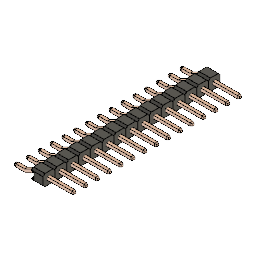
PinHeader_Male_RA_2.54mm (Autodesk Fusion 360 design; units mm, degrees)
part number: 2025-10-16-17-28-49-516
Autodesk Fusion 360 part; units mm, degrees
sketch "Sketch1" plane through (0, 0, 0) normal (0, 1, 0) x (1, 0, 0)
  line L0 (0, -0.64) -> (2.3, -0.64)
  line L1 (2.3, -0.64) -> (4.3, -1.59)
  line L2 (4.3, -1.59) -> (12.8, -1.59)
  line L3 (0, 0) -> (2.4443, 0)
  line L4 (2.4443, 0) -> (4.4443, -0.95)
  line L5 (4.4443, -0.95) -> (12.8, -0.95)
  line L6 (0, -0.64) -> (0, 0)
  line L7 (12.8, -1.59) -> (12.8, -0.95)
  line L8 (12.8, -1.27) -> (11.4, -1.27)
  dimension "d1" = 0.64
  dimension "d2" = 2.3
  dimension "d3" = 2
  dimension "d4" = 8.5
  dimension "d5" = -0.64
  dimension "d26" = 1.27
  constraint horizontal L0
  constraint parallel L0 L2
  constraint coincident L3.start L6.end
  constraint perpendicular L3 L6
  constraint perpendicular L2 L7
  constraint midpoint L7 L8.start
  constraint perpendicular L7 L8
  measures "d1" distance of L3.start L0.start
  measures "d2" distance of L0.start L0.end
  measures "d3" horizontal distance of L0.end L1.end
  measures "d4" distance of L1.end L2.end
  measures "d26" distance of L3.start L8
extrude "Extrude1" add sketch "Sketch1" along normal mid plane 0.64 makes body 1
sketch "Sketch2" plane through (0, 0, 0) normal (0, 1, 0) x (1, 0, 0)
  line L0 (4.7, -2.5) -> (7.2, -2.5)
  line L1 (7.2, -2.5) -> (7.2, 0)
  line L2 (7.2, 0) -> (4.7, 0)
  line L3 (4.7, 0) -> (4.7, -2.5)
  dimension "d9" = 2.5
  dimension "d10" = 4.7
  dimension "d11" = 2.5
  constraint horizontal L0
  constraint vertical L1
  constraint horizontal L2
  constraint vertical L3
  constraint coincident origin L2
  measures "d9" distance of L0.start L0.end
  measures "d10" distance of origin L3
  measures "d11" distance of L0.end L1.end
extrude "Extrude2" add sketch "Sketch2" along normal mid plane 2.54 separate body makes body 2
chamfer "Chamfer1" distance 0.1 angle 75 2 faces at (12.8, -0.1067, 1.3767) (0, 0.1067, 0.2133) on bodies 1
sketch "Sketch3" plane through (0, -1.27, 0) normal (0, -1, 0) x (1, 0, 0)
  line L0 (4.7, 2.5) -> (4.7, 0)
  line L1 (4.7, 0) -> (7.2, 0)
  line L2 (7.2, 0) -> (7.2, 2.5)
  line L3 (7.2, 2.5) -> (4.7, 2.5)
  line L4 (4.7, 1.9) -> (5.2, 1.9)
  line L5 (5.2, 1.9) -> (5.2, 0.6)
  line L6 (5.2, 0.6) -> (4.7, 0.6)
  line L7 (4.7, 0.6) -> (4.7, 1.9)
  line L8 (7.2, 1.25) -> (5.2, 1.25)
  dimension "d16" = 0.5
  dimension "d17" = 0.6
  constraint horizontal L4
  constraint vertical L5
  constraint horizontal L6
  constraint vertical L7
  constraint coincident L0 L4.start
  constraint midpoint L2 L8.start
  constraint midpoint L5 L8.end
  constraint horizontal L8
  measures "d16" distance of L4.start L4.end
  measures "d17" distance of L3 L4
extrude "Extrude3" cut sketch "Sketch3" against normal blind 2.6 contours L0 L4 L5 L6 L7 bodies 2
chamfer "Chamfer2" distance 0.4 angle 45 4 edges at (5.95, -1.27, 2.5) (5.95, 1.27, 2.5) (5.95, -1.27, 0) (5.95, 1.27, 0) on bodies 2
pattern_linear "R-Pattern1" count 15 spacing 2.54 along (0, 1, 0) of bodies 2 1 makes body 3 at (7.057, 2.86, 1.3767) makes body 4 at (7.2, 2.83, 0.8333) makes body 5 at (7.057, 5.4, 1.3767) makes body 6 at (7.2, 5.37, 0.8333) makes body 7 at (7.057, 7.94, 1.3767) makes body 8 at (7.2, 7.33, 1.6667) makes body 9 at (7.057, 10.48, 1.3767) makes body 10 at (7.2, 9.87, 1.6667) makes body 11 at (7.057, 13.02, 1.3767) makes body 12 at (7.2, 12.41, 1.6667) makes body 13 at (7.057, 15.56, 1.3767) makes body 14 at (7.2, 14.95, 1.6667) makes body 15 at (7.057, 18.1, 1.3767) makes body 16 at (7.2, 18.07, 1.6667) makes body 17 at (7.057, 20.64, 1.3767) makes body 18 at (7.2, 20.61, 1.6667) makes body 19 at (7.057, 23.18, 1.3767) makes body 20 at (7.2, 23.15, 1.6667) makes body 21 at (7.057, 25.72, 1.3767) makes body 22 at (7.2, 25.69, 1.6667) makes body 23 at (7.057, 28.26, 1.3767) makes body 24 at (7.2, 28.23, 1.6667) makes body 25 at (7.057, 30.8, 1.3767) makes body 26 at (7.2, 30.77, 1.6667) makes body 27 at (7.057, 33.34, 1.3767) makes body 28 at (7.2, 32.73, 1.6667) makes body 29 at (7.057, 35.88, 1.3767) makes body 30 at (7.2, 35.27, 1.6667)
equation "d4 = 2.5 mm + 6 mm"
equation "d10 = 1.8 mm + 2.9 mm"
equation "d21 = pins"
equation "pins = 15"
